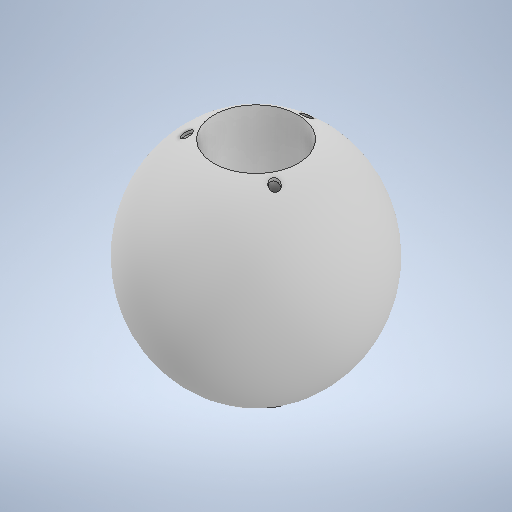
# Autodesk Inventor part: Buoy 9 SkinnySphere
Saved by Autodesk Inventor 2025 (Build 290162000, 162)
## iProperties
Created: 2024-07-03
Part Number: Buoy 9 SkinnySphere
Material: Generic
Document SubType Name: Modeling
Designer: track
Density: 1 g/cm^3
Appearance: Default
Mass: 900.619 g
Surface Area: 778.06 cm^2
Volume: 900.619 cm^3
Author: track
Autodesk Inventor part; units mm, degrees
ref_plane "YZ Plane" through (0, 0, 0) normal (1, 0, 0) x (0, 1, 0)
ref_plane "XZ Plane" through (0, 0, 0) normal (0, 1, 0) x (-1, 0, 0)
ref_plane "XY Plane" through (0, 0, 0) normal (0, 0, 1) x (1, 0, 0)
sketch "Sketch1" plane through (0, 0, 0) normal (0, 0, 1) x (1, 0, 0)
  line L0 (0, 0) -> (0, 127) construction
  line L1 (0, 0) -> (26.4, 0) construction
  line L2 (26.4, 0) -> (26.4, 127)
  arc A0 (26.4, 0) -> (26.4, 127) centre (-7.4667, 63.5) ccw
  line L3 (27.9, 124.4487) -> (27.9, 2.5513)
  arc A1 (27.9, 2.5513) -> (27.9, 124.4487) centre (-7.4667, 63.5) ccw
  point P0 (64.5, 63.5)
  dimension "d0" = 127
  dimension "d1" = 26.4
  dimension "d3" = 38.1
  dimension "d4" = 1.5
  constraints: 8 end point, 5 point on circle, 2 centre point, 1 horizontal, 1 perpendicular, 1 vertical, 1 other
  measures "d0" distance of L1.end L2.end
  measures "d1" distance of L0.start L1.end
  measures "d3" distance from line of L2 point (64.5, 63.5)
  measures "d4" distance between parallel lines of L2 L3
revolve "Revolution1" add sketch "Sketch1" angle 360 about axis through (0, 0, 0) along (0, 1, 0)
sketch "Sketch2" plane through (0, 0, 0) normal (0, 1, 0) x (-1, 0, 0)
  line L0 (0, 0) -> (0, -31.75) construction
  circle A0 centre (0, -31.75) radius 3
  dimension "d6" = 6
  dimension "d7" = 31.75
  constraints: 2 end point, 1 centre point, 1 coincident, 1 vertical
  measures "d6" diameter of A0
  measures "d7" distance of L0.start L0.end
extrude "Extrusion1" cut sketch "Sketch2" along normal through all
pattern_circular "Circular Pattern1" count 3 over 360 about axis through (0, 63.5, 0) along (0, 1, 0) of "Extrusion1"
body "Solid1"
